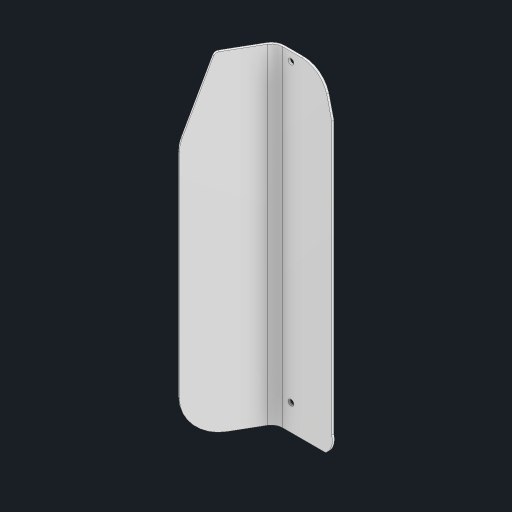
# Autodesk Inventor part: wedge
Saved by Autodesk Inventor 2024 (Build 280153000, 153)
## iProperties
Created: 2023-08-19
Part Number: wedge
Material: Acetal Resin, White
Document SubType Name: Modeling
Designer: Averey
Density: 1.425 g/cm^3
Appearance: Smooth - White
Author: Averey
Autodesk Inventor part; units mm, degrees
ref_plane "YZ Plane" through (0, 0, 0) normal (1, 0, 0) x (0, 1, 0)
ref_plane "XZ Plane" through (0, 0, 0) normal (0, 1, 0) x (-1, 0, 0)
ref_plane "XY Plane" through (0, 0, 0) normal (0, 0, 1) x (1, 0, 0)
sketch "Sketch1" plane through (0, 0, 0) normal (0, 0, 1) x (1, 0, 0)
  circle A0 centre (-3.1769, 113.7672) radius 2.0955
  circle A1 centre (-3.1769, -102.1328) radius 2.0955
  line L0 (-9.5269, 120.1172) -> (4.5684, 120.1172)
  line L1 (-9.5269, -121.1828) -> (-9.5269, 120.1172)
  line L2 (-9.5269, 120.1172) -> (-45.3591, 120.1172)
  line L3 (-66.6769, 60.3213) -> (-66.6769, -95.7828)
  line L4 (-9.5269, -121.1828) -> (-9.5269, 120.1172)
  line L5 (-48.3624, 117.9719) -> (-65.3039, 68.5592)
  arc A2 (-65.3039, 68.5592) -> (-66.6769, 60.3213) centre (-41.2769, 60.3213) ccw
  arc A3 (-66.6769, -95.7828) -> (-41.2769, -121.1828) centre (-41.2769, -95.7828) ccw
  arc A4 (-45.3591, 120.1172) -> (-48.3624, 117.9719) centre (-45.3591, 116.9422) ccw
  arc A5 (22.9235, 106.1658) -> (4.5684, 120.1172) centre (4.5684, 101.0672) ccw
  arc A6 (22.2231, -121.1828) -> (26.6067, -107.95) centre (14.337, -111.228) ccw
  line L6 (-41.2769, -121.1828) -> (22.2231, -121.1828)
  line L7 (26.6067, -107.95) -> (26.6067, 90.8579)
  line L8 (22.9235, 106.1658) -> (26.6067, 90.8579)
  point P0 (0, 0)
  point P1 (-66.6769, -121.1828)
  dimension "d0" = 4.191
  dimension "d1" = 4.191
  dimension "d2" = 57.15
  dimension "d3" = 25.4
  dimension "d4" = 3.175
  dimension "d5" = 19.05
  dimension "d16" = 12.7
  dimension "d18" = 63.5
  constraints: 18 end point, 10 point on circle, 7 centre point, 6 tangent, 3 horizontal, 2 point on line, 1 equal radius, 1 parallel, 1 perpendicular, 1 vertical
  measures "d0" diameter of A0
  measures "d1" diameter of A1
  measures "d2" distance of L1.start point (-66.677, -121.183)
  measures "d3" radius of A2
  measures "d4" radius of A4
  measures "d5" radius of A5
  measures "d16" radius of A6
  measures "d18" distance of L6.start L6.end
extrude "Extrusion1" add sketch "Sketch1" along normal blind 1.5875
bend part "Bend Part1" radius 9.525 angle 60 line through (-9.5269, -121.1828, 0) along (0, 1, 0) centre toward (0, 0, 1) moving side (-1, 0, 0) both sides no
body "Solid1"
